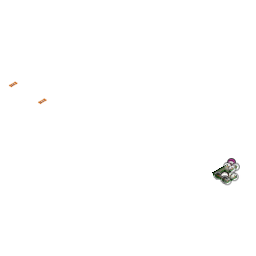
Y Axix Motor (Autodesk Fusion 360 design; units mm, degrees)
Autodesk Fusion 360 part; units mm, degrees
sketch "Skizze1" plane through (0, 0, 0) normal (0, 1, 0) x (1, 0, 0)
  ellipse E0 centre (19.0444, -49.1025) end of major axis (19.0444, -50.6334) minor radius 1.5307
  line L0 (55.2123, -43.6898) -> (55.2123, -85.3711)
  line L1 (55.2123, -85.3711) -> (13.531, -85.3711)
  line L2 (13.531, -85.3711) -> (13.531, -43.6898)
  line L3 (13.531, -43.6898) -> (55.2123, -43.6898)
  line L4 (26.9008, -1.7518) -> (30.0736, -4.9062)
  line L5 (30.0736, -4.9062) -> (30.0582, -31.0654)
  line L6 (30.0582, -31.0654) -> (30.1165, -31.0654)
  line L7 (30.1165, -31.0654) -> (30.1165, -42.123)
  line L8 (30.1165, -42.123) -> (63.94, -42.1236)
  line L9 (63.94, -42.1236) -> (67.115, -45.2984)
  line L10 (67.115, -45.2984) -> (67.115, -83.7656)
  line L11 (67.115, -83.7656) -> (63.94, -86.9404)
  line L12 (63.94, -86.9404) -> (4.096, -86.9404)
  line L13 (4.096, -86.9404) -> (0.9212, -83.7656)
  line L14 (0.9212, -83.7656) -> (0.9212, -4.9266)
  line L15 (0.9212, -4.9266) -> (4.0757, -1.7518)
  line L16 (4.0757, -1.7518) -> (26.9008, -1.7518)
  line L17 (-656.5386, -196.3597) -> (-656.5386, -172.9852) construction
  line L18 (-656.5386, -172.9852) -> (-663.2077, -172.9852) construction
  line L19 (-663.2077, -172.9852) -> (-663.2077, -196.3597) construction
  line L20 (-663.2077, -196.3597) -> (-656.5386, -196.3597) construction
  line L21 (-786.7672, -196.3598) -> (-786.7672, -172.9853) construction
  line L22 (-786.7672, -172.9853) -> (-793.4364, -172.9853) construction
  line L23 (-793.4364, -172.9853) -> (-793.4364, -196.3598) construction
  line L24 (-793.4364, -196.3598) -> (-786.7672, -196.3598) construction
  circle A0 centre (50.0444, -49.1025) radius 1.5 construction
  circle A1 centre (50.0444, -80.1025) radius 1.5 construction
  line L25 (50.0444, -80.1025) -> (19.0444, -80.1025) construction
  circle A2 centre (19.0444, -80.1025) radius 1.5 construction
  line L26 (19.0444, -80.1025) -> (19.0444, -49.1025) construction
  circle A3 centre (34.4717, -64.6752) radius 12.5 construction
  circle A4 centre (61.4704, -49.0847) radius 1.5 construction
  circle A5 centre (61.4704, -80.2249) radius 1.5 construction
  circle A6 centre (5.4074, -7.8253) radius 1.5 construction
  circle A7 centre (25.4061, -7.8253) radius 1.5 construction
  circle A8 centre (25.4061, -22.5328) radius 1.5 construction
  circle A9 centre (5.4074, -22.5328) radius 1.5 construction
  point P0 (51.8121, -49.1024)
  point P1 (51.6713, -79.7501)
  point P2 (19.0448, -81.2802)
  point P3 (19.0444, -50.6334)
  point P4 (34.1696, -76.3823)
  point P5 (27.8065, -7.8253)
  point P6 (27.8065, -22.5328)
  point P7 (7.8078, -7.8253)
  point P8 (7.8078, -22.5328)
  point P9 (10.9547, -80.1317)
  point P10 (10.9547, -48.9915)
  point P11 (63.8708, -80.2249)
  point P12 (63.8708, -49.0847)
  dimension "d1" = 31
  dimension "d2" = 3
  dimension "d4" = 3
  dimension "d5" = 31
  dimension "d6" = 3
  dimension "d7" = 25
  dimension "d8" = 3
  dimension "d9" = 3
  dimension "d10" = 3
  dimension "d11" = 3
  dimension "d12" = 3
  dimension "d13" = 3
  constraint coincident A1.centre L25.start
  constraint horizontal L25
  constraint coincident L25.end A2.centre
  constraint coincident E0.centre L26.end
  constraint perpendicular L25 L26
  measures "d1" distance of E0.centre A0.centre
  measures "d2" diameter of A0
  measures "d4" diameter of A1
  measures "d5" distance of A1.centre L25.end
  measures "d6" diameter of A2
  measures "d7" diameter of A3
  measures "d8" diameter of A4
  measures "d9" diameter of A5
  measures "d10" diameter of A6
  measures "d11" diameter of A7
  measures "d12" diameter of A8
  measures "d13" diameter of A9
extrude "Extrusion1" add sketch "Skizze1" along normal blind 4 contours L0 L1 L2 L3 | L4 L5 L6 L7 L8 L9 L10 L11 L12 L13 L14 L15 L16
sketch "Skizze2" plane through (0, 4, 0) normal (0, 1, 0) x (-1, 0, 0)
  ellipse E0 centre (-19.0444, 49.1025) end of major axis (-19.0444, 50.6334) minor radius 1.5307
  line L0 (-4.0757, 1.7518) -> (-0.9212, 4.9266)
  line L1 (-0.9212, 4.9266) -> (-0.9212, 83.7656)
  line L2 (-0.9212, 83.7656) -> (-4.096, 86.9404)
  line L3 (-4.096, 86.9404) -> (-63.94, 86.9404)
  line L4 (-63.94, 86.9404) -> (-67.115, 83.7656)
  line L5 (-67.115, 83.7656) -> (-67.115, 45.2984)
  line L6 (-67.115, 45.2984) -> (-63.94, 42.1236)
  line L7 (-63.94, 42.1236) -> (-30.1165, 42.123)
  line L8 (-30.1165, 42.123) -> (-30.1165, 31.0654)
  line L9 (-30.1165, 31.0654) -> (-30.0582, 31.0654)
  line L10 (-30.0582, 31.0654) -> (-30.0736, 4.9062)
  line L11 (-30.0736, 4.9062) -> (-26.9008, 1.7518)
  line L12 (-26.9008, 1.7518) -> (-4.0757, 1.7518)
  circle A0 centre (-50.0444, 49.1025) radius 1.5
  circle A1 centre (-50.0444, 80.1025) radius 1.5
  circle A2 centre (-19.0444, 80.1025) radius 1.5
  circle A3 centre (-34.5444, 64.6025) radius 12.5
  circle A4 centre (-5, 8) radius 1.5
  circle A5 centre (-25, 8) radius 1.5
  circle A6 centre (-5, 23) radius 1.5
  circle A7 centre (-25, 23) radius 1.5
  circle A8 centre (-63, 49) radius 1.5
  circle A9 centre (-63, 78) radius 1.5
  dimension "d16" = 31
  dimension "d17" = 3
  dimension "d18" = 31
  dimension "d19" = 3
  dimension "d20" = 31
  dimension "d21" = 3
  dimension "d22" = 25
  dimension "d23" = 3
  dimension "d24" = 3
  dimension "d25" = 3
  dimension "d26" = 15
  dimension "d27" = 3
  dimension "d28" = 3
  dimension "d29" = 3
  measures "d16" distance of E0.centre A0.centre
  measures "d17" diameter of A0
  measures "d18" distance of A0.centre A1.centre
  measures "d19" diameter of A1
  measures "d20" distance of A1.centre A2.centre
  measures "d21" diameter of A2
  measures "d22" diameter of A3
  measures "d23" diameter of A4
  measures "d24" diameter of A5
  measures "d25" diameter of A6
  measures "d26" distance of A5.centre A7.centre
  measures "d27" diameter of A7
  measures "d28" diameter of A8
  measures "d29" diameter of A9
extrude "Extrusion2" cut sketch "Skizze2" against normal blind 28 contours A0 | A1 | A2 | A3 | A4 | A5 | A6 | A7 | A8 | A9
sketch "Skizze3" plane through (0, 0, 0) normal (0, 1, 0) x (1, 0, 0)
